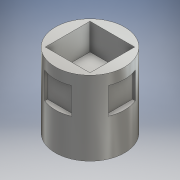
# Autodesk Inventor part: Enclosure
Saved by Autodesk Inventor 2016 (Build 200138000, 138)
## iProperties
Created: 2016-04-14
Part Number: Enclosure
Material: Generic
Document SubType Name: Modeling
Designer: Andres
Density: 1 g/cm^3
Appearance: Aluminum - Polished
Author: Andres
Autodesk Inventor part; units mm, degrees
ref_plane "YZ Plane" through (0, 0, 0) normal (1, 0, 0) x (0, 1, 0)
ref_plane "XZ Plane" through (0, 0, 0) normal (0, 1, 0) x (-1, 0, 0)
ref_plane "XY Plane" through (0, 0, 0) normal (0, 0, 1) x (1, 0, 0)
sketch "Sketch1" plane through (0, 0, 0) normal (0, 0, 1) x (1, 0, 0)
  circle A0 centre (0, 0) radius 32.5
  dimension "d32" = 65
  constraints: 1 centre point
  measures "d32" diameter of A0
extrude "Extrusion1" add sketch "Sketch1" along normal blind 70
sketch "Sketch2" plane through (0, 0, 70) normal (0, 0, 1) x (1, 0, 0)
  line L0 (-21, 21) -> (21, 21)
  line L1 (21, 21) -> (21, -21)
  line L2 (21, -21) -> (-21, -21)
  line L3 (-21, -21) -> (-21, 21)
  point P0 (0, 0)
  point P1 (-21, 0)
  point P2 (0, 21)
  dimension "d4" = 42
  dimension "d5" = 42
  constraints: 8 end point, 2 midpoint, 2 parallel, 1 horizontal, 1 horizontal alignment, 1 perpendicular, 1 vertical alignment
  measures "d4" distance of L0.end L1.end
  measures "d5" distance of L0.start L0.end
extrude "Extrusion2" cut sketch "Sketch2" against normal blind 25
sketch "Sketch3" plane through (0, 0, 45) normal (0, 0, 1) x (1, 0, 0)
  point P0 (0, 0)
sketch "Sketch4" plane through (0, 0, 0) normal (0, 0, -1) x (-1, 0, 0)
  circle A0 centre (0, 0) radius 5
  dimension "d8" = 10
  constraints: 1 centre point, 1 coincident
  measures "d8" diameter of A0
extrude "Extrusion3" cut sketch "Sketch4" against normal blind 10
sketch "Sketch5" plane through (0, 0, 10) normal (0, 0, -1) x (-1, 0, 0)
  circle A0 centre (0, 0) radius 2.5
  dimension "d11" = 5
  constraints: 1 centre point, 1 coincident
  measures "d11" diameter of A0
extrude "Extrusion4" cut sketch "Sketch5" against normal blind 35
sketch "Sketch6" plane through (0, 0, 0) normal (0, 0, -1) x (-1, 0, 0)
  line L0 (-7.5, -7.5) -> (7.5, -7.5)
  line L1 (7.5, -7.5) -> (7.5, 7.5)
  line L2 (7.5, 7.5) -> (-7.5, 7.5)
  line L3 (-7.5, 7.5) -> (-7.5, -7.5)
  point P0 (0, 0)
  point P1 (-7.5, 0)
  point P2 (0, 7.5)
  dimension "d14" = 15
  dimension "d15" = 15
  constraints: 8 end point, 2 midpoint, 2 parallel, 1 horizontal, 1 horizontal alignment, 1 perpendicular, 1 vertical alignment
  measures "d14" distance of L0.end L1.end
  measures "d15" distance of L0.start L0.end
extrude "Extrusion5" cut sketch "Sketch6" against normal blind 2.5
ref_plane "Work Plane2" through (0, 0, 10) normal (0, 0, -1) x (-1, 0, 0)
sketch "Sketch9" plane through (0, 0, 0) normal (0, 0, -1) x (-1, 0, 0)
  point P0 (0, 0)
ref_plane "Work Plane3" through (-21, 32.5, 70) normal (0, -1, 0) x (1, 0, 0)
sketch "Sketch11" plane through (-21, 32.5, 70) normal (0, -1, 0) x (1, 0, 0)
  line L0 (33.5, -10) -> (8.5, -10)
  line L1 (8.5, -10) -> (8.5, -35)
  line L2 (8.5, -35) -> (33.5, -35)
  line L3 (33.5, -35) -> (33.5, -10)
  line L4 (42, 0) -> (42, -25) projected
  line L5 (0, 0) -> (0, -25) projected
  line L6 (53.5, 0) -> (-11.5, 0) projected
  point P0 (21, -70)
  dimension "d34" = 25
  dimension "d35" = 25
  dimension "d36" = 8.5
  dimension "d37" = 8.5
  dimension "d38" = 10
  constraints: 8 end point, 2 parallel, 1 horizontal, 1 perpendicular
  measures "d34" distance of L0.end L1.end
  measures "d35" distance of L1.end L2.end
  measures "d36" distance between parallel lines of L3 L4
  measures "d37" distance between parallel lines of L1 L5
  measures "d38" distance between parallel lines of L6 L0
extrude "Extrusion6" cut sketch "Sketch11" along normal blind 5
ref_plane "Work Plane4" through (-21, -32.5, 70) normal (0, 1, 0) x (1, 0, 0)
ref_plane "Work Plane5" through (32.5, -21, 70) normal (-1, 0, 0) x (0, 0, 1)
ref_plane "Work Plane6" through (-32.5, -21, 70) normal (1, 0, 0) x (0, 0, -1)
sketch "Sketch12" plane through (-32.5, -21, 70) normal (1, 0, 0) x (0, 0, -1)
  line L0 (0, 53.5) -> (0, -11.5) projected
  line L1 (0, 42) -> (25, 42) projected
  line L2 (0, 0) -> (25, 0) projected
  line L3 (10, 33.5) -> (35, 33.5)
  line L4 (35, 33.5) -> (35, 8.5)
  line L5 (35, 8.5) -> (10, 8.5)
  line L6 (10, 8.5) -> (10, 33.5)
  point P0 (70, 21)
  dimension "d44" = 10
  dimension "d45" = 8.5
  dimension "d46" = 8.5
  dimension "d47" = 25
  constraints: 8 end point, 2 parallel, 1 horizontal, 1 perpendicular
  measures "d44" distance between parallel lines of L0 L6
  measures "d45" distance between parallel lines of L1 L3
  measures "d46" distance between parallel lines of L2 L5
  measures "d47" distance of L4.end L5.end
extrude "Extrusion7" cut sketch "Sketch12" along normal blind 5
sketch "Sketch13" plane through (-21, -32.5, 70) normal (0, 1, 0) x (1, 0, 0)
  line L0 (-11.5, 0) -> (53.5, 0) projected
  line L1 (0, 0) -> (0, 25) projected
  line L2 (42, 0) -> (42, 25) projected
  line L3 (8.5, 10) -> (33.5, 10)
  line L4 (33.5, 10) -> (33.5, 35)
  line L5 (33.5, 35) -> (8.5, 35)
  line L6 (8.5, 35) -> (8.5, 10)
  point P0 (21, 70)
  dimension "d50" = 10
  dimension "d51" = 8.5
  dimension "d52" = 8.5
  dimension "d53" = 25
  constraints: 8 end point, 2 parallel, 1 horizontal, 1 perpendicular
  measures "d50" distance between parallel lines of L0 L3
  measures "d51" distance between parallel lines of L1 L6
  measures "d52" distance between parallel lines of L2 L4
  measures "d53" distance of L3.end L4.end
extrude "Extrusion8" cut sketch "Sketch13" along normal blind 5
sketch "Sketch14" plane through (32.5, -21, 70) normal (-1, 0, 0) x (0, 0, 1)
  line L0 (0, -11.5) -> (0, 53.5) projected
  line L1 (0, 0) -> (-25, 0) projected
  line L2 (0, 42) -> (-25, 42) projected
  line L3 (-10, 8.5) -> (-35, 8.5)
  line L4 (-35, 8.5) -> (-35, 33.5)
  line L5 (-35, 33.5) -> (-10, 33.5)
  line L6 (-10, 33.5) -> (-10, 8.5)
  point P0 (-70, 21)
  dimension "d56" = 10
  dimension "d57" = 8.5
  dimension "d58" = 8.5
  dimension "d59" = 25
  constraints: 8 end point, 2 parallel, 1 horizontal, 1 perpendicular
  measures "d56" distance between parallel lines of L0 L6
  measures "d57" distance between parallel lines of L2 L5
  measures "d58" distance between parallel lines of L1 L3
  measures "d59" distance of L4.end L5.end
extrude "Extrusion9" cut sketch "Sketch14" along normal blind 5
body "Solid1"
